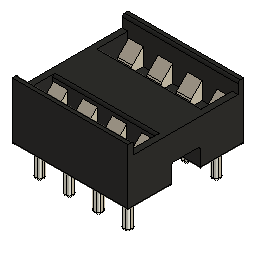
8_Pin_DIL (Autodesk Fusion 360 design; units mm, degrees)
Autodesk Fusion 360 part; units mm, degrees
sketch "Sketch1" plane through (0, 0, 0) normal (0, 0, 1) x (1, 0, 0)
  line L0 (5, -5) -> (-5, -5)
  line L1 (-5, -5) -> (-5, 5)
  line L2 (-5, 5) -> (5, 5)
  line L3 (5, 5) -> (5, -5)
  line L4 (5, -5) -> (-5, 5) construction
  line L5 (-5, -5) -> (5, 5) construction
  dimension "d1" = 10
  dimension "d2" = 10
  constraint horizontal L0
  constraint perpendicular L0 L1
  constraint parallel L0 L2
  constraint parallel L1 L3
  constraint coincident L4 origin
  constraint coincident L5 origin
  measures "d1" distance of L1.end L2.end
  measures "d2" distance of L0.end L1.end
extrude "Extrude1" add sketch "Sketch1" along normal blind 5
sketch "Sketch2" plane through (5, 0, 0) normal (1, 0, 0) x (0, 1, 0)
  line L0 (-5, 0) -> (5, 0)
  line L1 (5, 0) -> (5, 5)
  line L2 (5, 5) -> (-5, 5)
  line L3 (-5, 5) -> (-5, 0)
  line L4 (-1.25, 0) -> (1.25, 0)
  line L5 (1.25, 0) -> (1.25, 1.75)
  line L6 (1.25, 1.75) -> (-1.25, 1.75)
  line L7 (-1.25, 1.75) -> (-1.25, 0)
  line L8 (-5, 5) -> (-4.5, 5)
  line L9 (-4.5, 5) -> (-4.5, 4)
  line L10 (-4.5, 4) -> (-5, 4)
  line L11 (-5, 4) -> (-5, 5)
  line L12 (5, 5) -> (4.5, 5)
  line L13 (4.5, 5) -> (4.5, 4)
  line L14 (4.5, 4) -> (5, 4)
  line L15 (5, 4) -> (5, 5)
  line L16 (-4.5, 4) -> (4.5, 4)
  dimension "d5" = 2.5
  dimension "d6" = 1.75
  dimension "d7" = 3.75
  dimension "d10" = 0.5
  dimension "d11" = 1
  dimension "d12" = 0.5
  dimension "d13" = 1
  constraint horizontal L4
  constraint vertical L5
  constraint horizontal L6
  constraint vertical L7
  constraint coincident L0 L4.start
  constraint horizontal L8
  constraint vertical L9
  constraint horizontal L10
  constraint vertical L11
  constraint coincident L2.end L3.start
  constraint horizontal L12
  constraint vertical L13
  constraint horizontal L14
  constraint vertical L15
  constraint coincident L1.end L2.start
  measures "d5" distance of L4.start L4.end
  measures "d6" distance of L4.start L6.end
  measures "d7" distance of L1 L5
  measures "d10" distance of L2.end L8.end
  measures "d11" distance of L2.end L10.end
  measures "d12" distance of L1.end L12.end
  measures "d13" distance of L1.end L14.end
extrude "Extrude2" cut sketch "Sketch2" against normal blind 10 contours L0 L4 L5 L6 L7
extrude "Extrude3" cut sketch "Sketch2" against normal blind 10 contours L2 L9 L13 L16
sketch "Sketch3" plane through (0, 0, 4) normal (0, 0, 1) x (-1, 0, 0)
  line L0 (-5, 4.5) -> (-5, -4.5)
  line L1 (-5, -4.5) -> (5, -4.5)
  line L2 (5, -4.5) -> (5, 4.5)
  line L3 (5, 4.5) -> (-5, 4.5)
  line L4 (5, 2) -> (-5, 2)
  line L5 (-5, 2) -> (-5, -2)
  line L6 (-5, -2) -> (5, -2)
  line L7 (5, -2) -> (5, 2)
  line L8 (5, 4.5) -> (4.5, 4.5)
  line L9 (4.5, 4.5) -> (4.5, -4.5)
  line L10 (4.5, -4.5) -> (5, -4.5)
  line L11 (5, -4.5) -> (5, 4.5)
  line L12 (-5, -4.5) -> (-4.5, -4.5)
  line L13 (-4.5, -4.5) -> (-4.5, 4.5)
  line L14 (-4.5, 4.5) -> (-5, 4.5)
  line L15 (-5, 4.5) -> (-5, -4.5)
  dimension "d16" = 4
  dimension "d17" = 2.5
  dimension "d18" = 0.5
  dimension "d19" = 0.5
  constraint horizontal L4
  constraint vertical L5
  constraint horizontal L6
  constraint vertical L7
  constraint coincident L0 L5.end
  constraint coincident L2 L4.start
  constraint horizontal L8
  constraint vertical L9
  constraint horizontal L10
  constraint vertical L11
  constraint coincident L1 L9.end
  constraint coincident L2.end L3.start
  constraint horizontal L12
  constraint vertical L13
  constraint horizontal L14
  constraint vertical L15
  constraint coincident L3 L13.end
  constraint coincident L0.end L1.start
  measures "d16" distance of L4.start L6.end
  measures "d17" distance of L1 L6
  measures "d18" distance of L2.end L8.end
  measures "d19" distance of L0.end L12.end
extrude "Extrude4" cut sketch "Sketch3" against normal blind 2 contours L3 L4 L9 L13 | L1 L6 L9 L13
sketch "Sketch4" plane through (0, 0, 2) normal (0, 0, 1) x (-1, 0, 0)
  line L0 (4.5, 4.5) -> (-4.5, 4.5)
  line L1 (-4.5, 4.5) -> (-4.5, 2)
  line L2 (-4.5, 2) -> (4.5, 2)
  line L3 (4.5, 2) -> (4.5, 4.5)
  line L4 (-4.435, 4.5) -> (-3.185, 4.5)
  line L5 (-3.185, 4.5) -> (-3.185, 3.5)
  line L6 (-3.185, 3.5) -> (-4.435, 3.5)
  line L7 (-4.435, 3.5) -> (-4.435, 4.5)
  line L8 (-0.645, 4.5) -> (-0.645, 3.5)
  line L9 (-1.895, 4.5) -> (-0.645, 4.5)
  line L10 (-1.895, 3.5) -> (-1.895, 4.5)
  line L11 (-0.645, 3.5) -> (-1.895, 3.5)
  line L12 (1.895, 4.5) -> (1.895, 3.5)
  line L13 (0.645, 4.5) -> (1.895, 4.5)
  line L14 (0.645, 3.5) -> (0.645, 4.5)
  line L15 (1.895, 3.5) -> (0.645, 3.5)
  line L16 (4.435, 4.5) -> (4.435, 3.5)
  line L17 (3.185, 4.5) -> (4.435, 4.5)
  line L18 (3.185, 3.5) -> (3.185, 4.5)
  line L19 (4.435, 3.5) -> (3.185, 3.5)
  line L20 (-3.185, 3) -> (-3.185, 2)
  line L21 (-4.435, 3) -> (-3.185, 3)
  line L22 (-4.435, 2) -> (-4.435, 3)
  line L23 (-3.185, 2) -> (-4.435, 2)
  line L24 (-0.645, 3) -> (-0.645, 2)
  line L25 (-1.895, 3) -> (-0.645, 3)
  line L26 (-1.895, 2) -> (-1.895, 3)
  line L27 (-0.645, 2) -> (-1.895, 2)
  line L28 (1.895, 3) -> (1.895, 2)
  line L29 (0.645, 3) -> (1.895, 3)
  line L30 (0.645, 2) -> (0.645, 3)
  line L31 (1.895, 2) -> (0.645, 2)
  line L32 (4.435, 3) -> (4.435, 2)
  line L33 (3.185, 3) -> (4.435, 3)
  line L34 (3.185, 2) -> (3.185, 3)
  line L35 (4.435, 2) -> (3.185, 2)
  dimension "d22" = 1.25
  dimension "d23" = 1
  dimension "d26" = -2.54
  dimension "d27" = 1.5
  dimension "d28" = 0.065
  constraint horizontal L4
  constraint vertical L5
  constraint horizontal L6
  constraint vertical L7
  constraint coincident L4.start
  measures "d22" distance of L4.start L4.end
  measures "d23" distance of L4.start L6.end
  measures "d28" distance of L1 L7
extrude "Extrude5" add sketch "Sketch4" along normal blind 1.5 contours L0 L16 L17 L18 L19 | L2 L32 L33 L34 L35 | L0 L12 L13 L14 L15 | L2 L28 L29 L30 L31 | L0 L8 L9 L10 L11 | L2 L24 L25 L26 L27 | L0 L4 L5 L6 L7 | L2 L20 L21 L22 L23
chamfer "Chamfer1" distance 1 angle 45 8 edges at (-1.27, -3.5, 3.5) (-3.81, -3.5, 3.5) (-3.81, -3, 3.5) (-1.27, -3, 3.5) (1.27, -3.5, 3.5) (1.27, -3, 3.5) (3.81, -3.5, 3.5) (3.81, -3, 3.5)
mirror "Mirror1" about plane through (0, 0, 0) normal (0, 1, 0) of "Extrude5", "Chamfer1"
fillet "Fillet1" radius 0.2 22 edges at (0, -1.25, 1.75) (0, 1.25, 1.75) (0, -4.5, 5) (0, 4.5, 5) (0, 2, 4) (0, -2, 4) (-3.81, -3.5, 2.5) (-3.81, -3, 2.5) (-1.27, -3.5, 2.5) (-1.27, -3, 2.5) (1.27, -3.5, 2.5) (1.27, -3, 2.5) (3.81, -3.5, 2.5) (3.81, -3, 2.5) (3.81, 3, 2.5) (3.81, 3.5, 2.5) (1.27, 3.5, 2.5) (1.27, 3, 2.5) (-1.27, 3, 2.5) (-1.27, 3.5, 2.5) (-3.81, 3.5, 2.5) (-3.81, 3, 2.5) 2 faces at (-1.6667, -3.75, 0) (-1.6667, 2.5, 0)
sketch "Sketch5" plane through (0, 0, 0) normal (0, 0, -1) x (1, 0, 0)
  line L0 (-4.8, -4.8) -> (4.8, -4.8)
  line L1 (4.8, -4.8) -> (4.8, -1.45)
  line L2 (4.8, -1.45) -> (-4.8, -1.45)
  line L3 (-4.8, -1.45) -> (-4.8, -4.8)
  line L4 (3.185, -3) -> (4.435, -3)
  line L5 (4.435, -3) -> (3.185, -3)
  line L6 (4.435, -3.5) -> (3.185, -3.5)
  line L7 (3.185, -3.5) -> (4.435, -3.5)
  line L8 (3.485, -3.4875) -> (4.135, -3.4875)
  line L9 (4.135, -3.4875) -> (4.135, -4.1375)
  line L10 (4.135, -4.1375) -> (3.485, -4.1375)
  line L11 (3.485, -4.1375) -> (3.485, -3.4875)
  line L12 (3.485, -3.4875) -> (4.135, -4.1375) construction
  line L13 (4.135, -3.4875) -> (3.485, -4.1375) construction
  line L14 (3.81, -4.0625) -> (3.81, -3.5625)
  line L15 (3.81, -3.8125) -> (3.185, -3.5)
  point P0 (3.81, -3.8125)
  dimension "d36" = 0.65
  dimension "d37" = 0.65
  dimension "d48" = 0.99
  constraint horizontal L8
  constraint perpendicular L8 L9
  constraint parallel L8 L10
  constraint parallel L9 L11
  constraint coincident L12 P0
  constraint coincident L13 P0
  constraint midpoint L14 P0
  constraint coincident L6.end L7.start
  constraint coincident P0 L15.start
  measures "d36" distance of L9.end L10.end
  measures "d37" distance of L8.end L9.end
  measures "d48" distance of L1 L14
extrude "Extrude6" add sketch "Sketch5" along normal blind 2.5 contours L6 L7 L9 L10 L11 | L6 L7 L8 L9 L11
fillet "Fillet2" radius 0.2 4 edges at (4.135, 4.1375, -1.25) (3.485, 4.1375, -1.25) (4.135, 3.4875, -1.25) (3.485, 3.4875, -1.25) 1 faces at (3.7017, 3.7042, -2.5)
pattern_linear "R-Pattern1" count 4 spacing 2.54 along (-1, 0, 0) of "Extrude6", "Fillet2"
mirror "Mirror2" about plane through (0, 0, 0) normal (0, 1, 0) of "Extrude6", "Fillet2", "R-Pattern1"
equation "d7 = ( 7.5 / 2 ) * 1 mm"
named bodies: "8-Pin_DIL"
